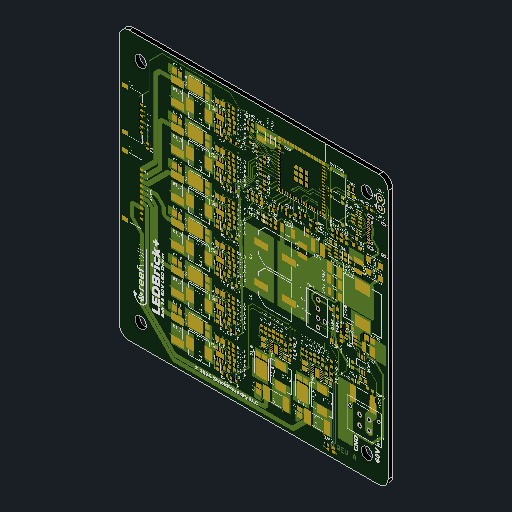
# Autodesk Inventor part: rv_ledbrick_8ch_BOARD
Saved by Autodesk Inventor 2026.1 (Build 301233020, 233B)
## iProperties
Created: 2025-09-11
Part Number: rv_ledbrick_8ch_BOARD
Material: Generic
Document SubType Name: Modeling
Designer: atrus
Density: 1 g/cm^3
Appearance: BoardColor
Author: atrus
Autodesk Inventor part; units mm, degrees
ref_plane "YZ Plane" through (0, 0, 0) normal (1, 0, 0) x (0, 1, 0)
ref_plane "XZ Plane" through (0, 0, 0) normal (0, 1, 0) x (-1, 0, 0)
ref_plane "BoardFrontPlane" through (0, 0, 0) normal (0, 0, 1) x (1, 0, 0)
sketch "Sketch1" plane through (0, 0, 0) normal (0, 0, 1) x (1, 0, 0)
  line L0 (30, 30) -> (30, 109)
  arc A0 (33, 112) -> (30, 109) centre (33, 109) ccw
  line L1 (33, 112) -> (112, 112)
  arc A1 (115, 109) -> (112, 112) centre (112, 109) ccw
  line L2 (115, 109) -> (115, 30)
  arc A2 (112, 27) -> (115, 30) centre (112, 30) ccw
  line L3 (112, 27) -> (33, 27)
  arc A3 (30, 30) -> (33, 27) centre (33, 30) ccw
  constraints: 8 end point, 8 point on circle, 4 centre point
extrude "BoardOutline" add sketch "Sketch1" along normal blind 1.4202
sketch "img_Top" plane through (0, 0, 1.4202) normal (0, 0, 1) x (1, 0, 0)
  line L0 (30, 112) -> (115, 112) construction
  line L1 (115, 112) -> (115, 27) construction
  line L2 (115, 27) -> (30, 27) construction
  line L3 (30, 27) -> (30, 112) construction
  constraints: 2 other
decal "Decal_Top"
sketch "img_Bottom" plane through (0, 0, -1.4202) normal (0, 0, -1) x (1, 0, 0)
  line L0 (30, -27) -> (115, -27) construction
  line L1 (115, -27) -> (115, -112) construction
  line L2 (115, -112) -> (30, -112) construction
  line L3 (30, -112) -> (30, -27) construction
  constraints: 2 other
decal "Decal_Bottom"
sketch "Sketch4" plane through (0, 0, 1.4202) normal (0, 0, 1) x (1, 0, 0)
  point P0 (111.97, 44.138)
hole "J500-_KOGJUJYS" at (111.97, 44.138, 1.4202) direction (0, 0, -1) diameter 1.02 end through all
sketch "Sketch5" plane through (0, 0, 1.4202) normal (0, 0, 1) x (1, 0, 0)
  point P0 (102.97, 44.138)
hole "J500-_FQXDTYVQ" at (102.97, 44.138, 1.4202) direction (0, 0, -1) diameter 1.02 end through all
sketch "Sketch6" plane through (0, 0, 1.4202) normal (0, 0, 1) x (1, 0, 0)
  point P0 (105.97, 43.198)
hole "J500-4" at (105.97, 43.198, 1.4202) direction (0, 0, -1) diameter 1.02 end through all
sketch "Sketch7" plane through (0, 0, 1.4202) normal (0, 0, 1) x (1, 0, 0)
  point P0 (108.97, 43.198)
hole "J500-3" at (108.97, 43.198, 1.4202) direction (0, 0, -1) diameter 1.02 end through all
sketch "Sketch8" plane through (0, 0, 1.4202) normal (0, 0, 1) x (1, 0, 0)
  point P0 (105.97, 40.198)
hole "J500-2" at (105.97, 40.198, 1.4202) direction (0, 0, -1) diameter 1.02 end through all
sketch "Sketch9" plane through (0, 0, 1.4202) normal (0, 0, 1) x (1, 0, 0)
  point P0 (108.97, 40.198)
hole "J500-1" at (108.97, 40.198, 1.4202) direction (0, 0, -1) diameter 1.02 end through all
sketch "Sketch10" plane through (0, 0, 1.4202) normal (0, 0, 1) x (1, 0, 0)
  point P0 (92.84, 68.08)
hole "J201-1" at (92.84, 68.08, 1.4202) direction (0, 0, -1) diameter 1.02 end through all
sketch "Sketch11" plane through (0, 0, 1.4202) normal (0, 0, 1) x (1, 0, 0)
  point P0 (92.84, 65.54)
  dimension "d25" = 25.4
hole "J201-2" at (92.84, 65.54, 1.4202) direction (0, 0, -1) diameter 1.02 end through all
sketch "Sketch12" plane through (0, 0, 1.4202) normal (0, 0, 1) x (1, 0, 0)
  point P0 (92.84, 63)
hole "J201-3" at (92.84, 63, 1.4202) direction (0, 0, -1) diameter 1.02 end through all
sketch "Sketch13" plane through (0, 0, 1.4202) normal (0, 0, 1) x (1, 0, 0)
  point P0 (92.84, 60.46)
hole "J201-4" at (92.84, 60.46, 1.4202) direction (0, 0, -1) diameter 1.02 end through all
sketch "Sketch14" plane through (0, 0, 1.4202) normal (0, 0, 1) x (1, 0, 0)
  point P0 (95, 63)
hole "J201-GUIDE" at (95, 63, 1.4202) direction (0, 0, -1) diameter 1.25 end through all
sketch "Sketch15" plane through (0, 0, 1.4202) normal (0, 0, 1) x (1, 0, 0)
  line L0 (109.936, 90.498) -> (108.836, 90.498) construction
  line L1 (109.936, 90.798) -> (108.836, 90.798)
  line L2 (108.836, 90.198) -> (109.936, 90.198)
  arc A0 (109.936, 90.198) -> (109.936, 90.798) centre (109.936, 90.498) ccw
  arc A1 (108.836, 90.798) -> (108.836, 90.198) centre (108.836, 90.498) ccw
  point P0 (109.386, 90.498)
  constraints: 8 end point, 4 point on circle, 4 tangent, 2 centre point, 1 midpoint, 1 parallel
extrude "J300-SH1" cut sketch "Sketch15" against normal through all
sketch "Sketch16" plane through (0, 0, 1.4202) normal (0, 0, 1) x (1, 0, 0)
  line L0 (109.936, 99.138) -> (108.836, 99.138) construction
  line L1 (109.936, 99.438) -> (108.836, 99.438)
  line L2 (108.836, 98.838) -> (109.936, 98.838)
  arc A0 (109.936, 98.838) -> (109.936, 99.438) centre (109.936, 99.138) ccw
  arc A1 (108.836, 99.438) -> (108.836, 98.838) centre (108.836, 99.138) ccw
  point P0 (109.386, 99.138)
  constraints: 8 end point, 4 point on circle, 4 tangent, 2 centre point, 1 midpoint, 1 parallel
extrude "J300-SH2" cut sketch "Sketch16" against normal through all
sketch "Sketch17" plane through (0, 0, 1.4202) normal (0, 0, 1) x (1, 0, 0)
  line L0 (113.966, 90.498) -> (113.166, 90.498) construction
  line L1 (113.966, 90.798) -> (113.166, 90.798)
  line L2 (113.166, 90.198) -> (113.966, 90.198)
  arc A0 (113.966, 90.198) -> (113.966, 90.798) centre (113.966, 90.498) ccw
  arc A1 (113.166, 90.798) -> (113.166, 90.198) centre (113.166, 90.498) ccw
  point P0 (113.566, 90.498)
  constraints: 8 end point, 4 point on circle, 4 tangent, 2 centre point, 1 midpoint, 1 parallel
extrude "J300-SH3" cut sketch "Sketch17" against normal through all
sketch "Sketch18" plane through (0, 0, 1.4202) normal (0, 0, 1) x (1, 0, 0)
  line L0 (113.966, 99.138) -> (113.166, 99.138) construction
  line L1 (113.966, 99.438) -> (113.166, 99.438)
  line L2 (113.166, 98.838) -> (113.966, 98.838)
  arc A0 (113.966, 98.838) -> (113.966, 99.438) centre (113.966, 99.138) ccw
  arc A1 (113.166, 99.438) -> (113.166, 98.838) centre (113.166, 99.138) ccw
  point P0 (113.566, 99.138)
  constraints: 8 end point, 4 point on circle, 4 tangent, 2 centre point, 1 midpoint, 1 parallel
extrude "J300-SH4" cut sketch "Sketch18" against normal through all
sketch "Sketch19" plane through (0, 0, 1.4202) normal (0, 0, 1) x (1, 0, 0)
  point P0 (109.886, 97.708)
hole "J300-_CAEUAXLF" at (109.886, 97.708, 1.4202) direction (0, 0, -1) diameter 0.65 end through all
sketch "Sketch20" plane through (0, 0, 1.4202) normal (0, 0, 1) x (1, 0, 0)
  point P0 (109.886, 91.928)
hole "J300-_KDPGCBUA" at (109.886, 91.928, 1.4202) direction (0, 0, -1) diameter 0.65 end through all
sketch "Sketch21" plane through (0, 0, 1.4202) normal (0, 0, 1) x (1, 0, 0)
  point P0 (108.25, 105.25)
hole "Free-5" at (108.25, 105.25, 1.4202) direction (0, 0, -1) diameter 3.6 end through all
sketch "Sketch22" plane through (0, 0, 1.4202) normal (0, 0, 1) x (1, 0, 0)
  point P0 (108.25, 33.75)
hole "Free-4" at (108.25, 33.75, 1.4202) direction (0, 0, -1) diameter 3.6 end through all
sketch "Sketch23" plane through (0, 0, 1.4202) normal (0, 0, 1) x (1, 0, 0)
  point P0 (36.75, 105.25)
hole "Free-3" at (36.75, 105.25, 1.4202) direction (0, 0, -1) diameter 3.6 end through all
sketch "Sketch24" plane through (0, 0, 1.4202) normal (0, 0, 1) x (1, 0, 0)
  point P0 (36.75, 33.75)
hole "Free-2" at (36.75, 33.75, 1.4202) direction (0, 0, -1) diameter 3.6 end through all
sketch "Sketch25" plane through (0, 0, 1.4202) normal (0, 0, 1) x (1, 0, 0)
  line L0 (45.048, 97) -> (71, 97)
  line L1 (71, 97) -> (71, 110)
  line L2 (71, 110) -> (45.048, 110)
  line L3 (45.048, 110) -> (45.048, 97)
  constraints: 8 end point
surface extrude "A" sketch "Sketch25" along normal blind 0.0508 shown yes curves L0 L1 L2 L3
sketch "Sketch26" plane through (0, 0, 1.4202) normal (0, 0, 1) x (1, 0, 0)
  line L0 (69.342, 27.686) -> (114.3, 27.686)
  line L1 (114.3, 27.686) -> (114.3, 112.776)
  line L2 (114.3, 112.776) -> (69.342, 112.776)
  line L3 (69.342, 112.776) -> (69.342, 27.686)
  constraints: 8 end point
surface extrude "U_rv_ledbrick_logic" sketch "Sketch26" along normal blind 0.0508 shown yes curves L0 L1 L2 L3
sketch "Sketch27" plane through (0, 0, 1.4202) normal (0, 0, 1) x (1, 0, 0)
  line L0 (45.048, 32) -> (71, 32)
  line L1 (71, 32) -> (71, 45)
  line L2 (71, 45) -> (45.048, 45)
  line L3 (45.048, 45) -> (45.048, 32)
  constraints: 8 end point
surface extrude "F" sketch "Sketch27" along normal blind 0.0508 shown yes curves L0 L1 L2 L3
sketch "Sketch28" plane through (0, 0, 1.4202) normal (0, 0, 1) x (1, 0, 0)
  line L0 (45.048, 71) -> (71, 71)
  line L1 (71, 71) -> (71, 84)
  line L2 (71, 84) -> (45.048, 84)
  line L3 (45.048, 84) -> (45.048, 71)
  constraints: 8 end point
surface extrude "C" sketch "Sketch28" along normal blind 0.0508 shown yes curves L0 L1 L2 L3
sketch "Sketch29" plane through (0, 0, 1.4202) normal (0, 0, 1) x (1, 0, 0)
  line L0 (45.048, 84) -> (71, 84)
  line L1 (71, 84) -> (71, 97)
  line L2 (71, 97) -> (45.048, 97)
  line L3 (45.048, 97) -> (45.048, 84)
  constraints: 8 end point
surface extrude "B" sketch "Sketch29" along normal blind 0.0508 shown yes curves L0 L1 L2 L3
sketch "Sketch30" plane through (0, 0, 1.4202) normal (0, 0, 1) x (1, 0, 0)
  line L0 (45.048, 58) -> (71, 58)
  line L1 (71, 58) -> (71, 71)
  line L2 (71, 71) -> (45.048, 71)
  line L3 (45.048, 71) -> (45.048, 58)
  constraints: 8 end point
surface extrude "D" sketch "Sketch30" along normal blind 0.0508 shown yes curves L0 L1 L2 L3
sketch "Sketch31" plane through (0, 0, 1.4202) normal (0, 0, 1) x (1, 0, 0)
  line L0 (45.048, 45) -> (71, 45)
  line L1 (71, 45) -> (71, 58)
  line L2 (71, 58) -> (45.048, 58)
  line L3 (45.048, 58) -> (45.048, 45)
  constraints: 8 end point
surface extrude "E" sketch "Sketch31" along normal blind 0.0508 shown yes curves L0 L1 L2 L3
sketch "Sketch32" plane through (0, 0, 1.4202) normal (0, 0, 1) x (1, 0, 0)
  line L0 (98, 31.048) -> (98, 57)
  line L1 (98, 57) -> (85, 57)
  line L2 (85, 57) -> (85, 31.048)
  line L3 (85, 31.048) -> (98, 31.048)
  constraints: 8 end point
surface extrude "H" sketch "Sketch32" along normal blind 0.0508 shown yes curves L0 L1 L2 L3
sketch "Sketch33" plane through (0, 0, 1.4202) normal (0, 0, 1) x (1, 0, 0)
  line L0 (85, 31) -> (85, 56.952)
  line L1 (85, 56.952) -> (72, 56.952)
  line L2 (72, 56.952) -> (72, 31)
  line L3 (72, 31) -> (85, 31)
  constraints: 8 end point
surface extrude "G" sketch "Sketch33" along normal blind 0.0508 shown yes curves L0 L1 L2 L3
sketch "Sketch34" plane through (0, 0, 1.4202) normal (0, 0, 1) x (1, 0, 0)
  line L0 (80.264, 59.182) -> (113.792, 59.182)
  line L1 (113.792, 59.182) -> (113.792, 88.9)
  line L2 (113.792, 88.9) -> (80.264, 88.9)
  line L3 (80.264, 88.9) -> (80.264, 59.182)
  constraints: 8 end point
surface extrude "U_dcdc_60v_12v" sketch "Sketch34" along normal blind 0.0508 shown yes curves L0 L1 L2 L3
sketch "Sketch35" plane through (0, 0, 1.4202) normal (0, 0, 1) x (1, 0, 0)
  line L0 (101.6, 89.408) -> (116.84, 89.408)
  line L1 (116.84, 89.408) -> (116.84, 100.584)
  line L2 (116.84, 100.584) -> (101.6, 100.584)
  line L3 (101.6, 100.584) -> (101.6, 89.408)
  constraints: 8 end point
surface extrude "U_usb_input" sketch "Sketch35" along normal blind 0.0508 shown yes curves L0 L1 L2 L3
sketch "Sketch36" plane through (0, 0, 1.4202) normal (0, 0, 1) x (1, 0, 0)
  line L0 (101.473, 36.957) -> (114.046, 36.957)
  line L1 (114.046, 36.957) -> (114.046, 61.595)
  line L2 (114.046, 61.595) -> (101.473, 61.595)
  line L3 (101.473, 61.595) -> (101.473, 36.957)
  constraints: 8 end point
surface extrude "U_vin_shunt" sketch "Sketch36" along normal blind 0.0508 shown yes curves L0 L1 L2 L3
sketch "Sketch37" plane through (0, 0, 1.4202) normal (0, 0, 1) x (1, 0, 0)
  point P0 (112.5, 105.5)
hole "J200-2" at (112.5, 105.5, 1.4202) direction (0, 0, -1) diameter 1.016 end through all
sketch "Sketch38" plane through (0, 0, 1.4202) normal (0, 0, 1) x (1, 0, 0)
  point P0 (112.5, 102.96)
hole "J200-1" at (112.5, 102.96, 1.4202) direction (0, 0, -1) diameter 1.016 end through all
body "Solid1"
body "Srf1"
body "Srf2"
body "Srf3"
body "Srf4"
body "Srf5"
body "Srf6"
body "Srf7"
body "Srf8"
body "Srf9"
body "Srf10"
body "Srf11"
body "Srf12"
